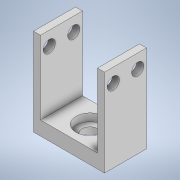
# Autodesk Inventor part: magnetsupport
Saved by Autodesk Inventor 2022 (Build 260153000, 153)
## iProperties
Created: 2022-08-13
Part Number: magnetsupport
Material: Genérico
Document SubType Name: Modeling
Designer: JK
Density: 1 g/cm^3
Appearance: Valor por defecto
Author: JK
Autodesk Inventor part; units mm, degrees
ref_plane "YZ Plane" through (0, 0, 0) normal (1, 0, 0) x (0, 1, 0)
ref_plane "XZ Plane" through (0, 0, 0) normal (0, 1, 0) x (-1, 0, 0)
ref_plane "XY Plane" through (0, 0, 0) normal (0, 0, 1) x (1, 0, 0)
sketch "Boceto1" plane through (0, 0, 0) normal (0, 1, 0) x (-1, 0, 0)
  circle A0 centre (0, 0) radius 2.25
  line L0 (-8.15, 6) -> (8.15, 6)
  line L1 (8.15, 6) -> (8.15, -6)
  line L2 (8.15, -6) -> (-8.15, -6)
  line L3 (-8.15, -6) -> (-8.15, 6)
  line L4 (-8.15, 6) -> (8.15, -6) construction
  line L5 (8.15, 6) -> (-8.15, -6) construction
  dimension "d0" = 4.5
  dimension "d1" = 16.3
  dimension "d2" = 12
  constraints: 12 end point, 2 midpoint, 2 parallel, 1 centre point, 1 coincident, 1 horizontal, 1 perpendicular
  measures "d0" diameter of A0
  measures "d1" distance of L1.end L2.end
  measures "d2" distance of L0.end L1.end
extrude "Extrusión1" add sketch "Boceto1" along normal blind 4
sketch "Boceto2" plane through (0, 4, 0) normal (0, 1, 0) x (1, 0, 0)
  circle A0 centre (0, 0) radius 4
  dimension "d5" = 8
  constraints: 1 centre point, 1 coincident
  measures "d5" diameter of A0
extrude "Extrusión2" cut sketch "Boceto2" against normal blind 2.2
sketch "Boceto3" plane through (0, 0, 0) normal (0, -1, 0) x (1, 0, 0)
  line L0 (10.15, 6) -> (-10.15, 6)
  line L1 (-10.15, 6) -> (-10.15, -6)
  line L2 (-10.15, -6) -> (10.15, -6)
  line L3 (10.15, -6) -> (10.15, 6)
  circle A0 centre (0, 0) radius 2.25 projected
  line L4 (10.15, 6) -> (-10.15, -6) construction
  line L5 (-10.15, 6) -> (10.15, -6) construction
  line L6 (8.15, -6) -> (-8.15, -6) projected
  line L7 (8.15, 6) -> (8.15, -6) projected
  line L8 (8.15, -6) -> (-8.15, -6) projected
  line L9 (8.15, 6) -> (8.15, -6) projected
  line L10 (-8.15, 6) -> (8.15, 6) projected
  line L11 (-8.15, -6) -> (-8.15, 6) projected
  circle A1 centre (0, 0) radius 2.25 projected
  point P0 (8.15, -6)
  point P1 (-8.15, -6)
  point P2 (-8.15, 6)
  dimension "d8" = 2
  constraints: 12 end point, 2 midpoint, 2 parallel, 1 collinear, 1 horizontal, 1 perpendicular
  measures "d8" distance between parallel lines of L7 L3
extrude "Extrusión3" add sketch "Boceto3" against normal blind 25 contours L3 L2 L7 L0 | L11 L2 L1 L0
sketch "Boceto4" plane through (10.15, 0, 6) normal (1, 0, 0) x (0, 0, -1)
  circle A0 centre (2.5, 21) radius 1.75
  circle A1 centre (9.5, 21) radius 1.75
  line L0 (0, 25) -> (12, 25) projected
  line L1 (0, 0) -> (0, 25) projected
  point P0 (6, 0)
  dimension "d11" = 4
  dimension "d12" = 3.5
  dimension "d14" = 7
  dimension "d15" = 2.5
  constraints: 2 centre point, 1 equal radius, 1 horizontal alignment
  measures "d11" distance from line of L0 A1.centre
  measures "d12" diameter of A1
  measures "d14" distance of A1.centre A0.centre
  measures "d15" distance from line of L1 A0.centre
extrude "Extrusión4" cut sketch "Boceto4" against normal through all
